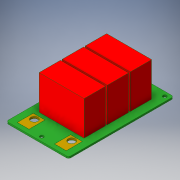
# Autodesk Inventor part: Cap_Platine
Saved by Autodesk Inventor 2016 (Build 200138000, 138)
## iProperties
Created: 2018-04-27
Part Number: Cap_Platine
Material: Generic
Document SubType Name: Modeling
Designer: Phil Erle
Density: 1 g/cm^3
Appearance: Smooth - Dark Forest Green
Author: Phil Erle
Autodesk Inventor part; units mm, degrees
ref_plane "YZ Plane" through (0, 0, 0) normal (1, 0, 0) x (0, 1, 0)
ref_plane "XZ Plane" through (0, 0, 0) normal (0, 1, 0) x (-1, 0, 0)
ref_plane "XY Plane" through (0, 0, 0) normal (0, 0, 1) x (1, 0, 0)
sketch "Sketch1" plane through (0, 0, 0) normal (0, 0, 1) x (1, 0, 0)
  line L0 (-29, -49) -> (29, -49)
  line L1 (29, -49) -> (29, 49)
  line L2 (29, 49) -> (-29, 49)
  line L3 (-29, 49) -> (-29, -49)
  line L4 (-29, -49) -> (29, 49) construction
  line L5 (29, -49) -> (-29, 49) construction
  point P0 (0, 0)
  dimension "d0" = 58
  dimension "d1" = 98
  constraints: 12 end point, 2 midpoint, 2 parallel, 1 horizontal, 1 perpendicular
  measures "d0" distance of L2.end L1.end
  measures "d1" distance of L1.end L0.end
extrude "Extrusion1" add sketch "Sketch1" along normal blind 1.6
sketch "Sketch2" plane through (0, 0, 1.6) normal (0, 0, 1) x (1, 0, 0)
  line L0 (-21, 16.5) -> (21, 16.5)
  line L1 (21, 16.5) -> (21, 36.5)
  line L2 (21, 36.5) -> (-21, 36.5)
  line L3 (-21, 36.5) -> (-21, 16.5)
  line L4 (-21, 16.5) -> (21, 36.5) construction
  line L5 (21, 16.5) -> (-21, 36.5) construction
  line L6 (-21, -5) -> (21, -5)
  line L7 (21, -5) -> (21, 15)
  line L8 (21, 15) -> (-21, 15)
  line L9 (-21, 15) -> (-21, -5)
  line L10 (-21, -5) -> (21, 15) construction
  line L11 (21, -5) -> (-21, 15) construction
  line L12 (-21, -26.5) -> (21, -26.5)
  line L13 (21, -26.5) -> (21, -6.5)
  line L14 (21, -6.5) -> (-21, -6.5)
  line L15 (-21, -6.5) -> (-21, -26.5)
  line L16 (-21, -26.5) -> (21, -6.5) construction
  line L17 (21, -26.5) -> (-21, -6.5) construction
  line L18 (-29, -49) -> (29, -49) projected
  line L19 (29, 49) -> (-29, 49) projected
  point P0 (0, 0)
  point P1 (0, 26.5)
  point P2 (0, 5)
  point P3 (0, -16.5)
  point P4 (0, 16.5)
  dimension "d4" = 42
  dimension "d5" = 20
  dimension "d6" = 20
  dimension "d7" = 20
  dimension "d8" = 1.5
  dimension "d9" = 1.5
  dimension "d31" = 12.5
  constraints: 36 end point, 7 midpoint, 6 parallel, 5 vertical alignment, 3 horizontal, 3 perpendicular
  measures "d4" distance of L1.end L2.end
  measures "d5" distance of L0.end L1.end
  measures "d6" distance of L6.end L7.end
  measures "d7" distance of L12.end L13.end
  measures "d8" distance of L13.end L6.end
  measures "d9" distance of L7.end L0.end
  measures "d31" distance between parallel lines of L19 L2
extrude "Extrusion2" add sketch "Sketch2" along normal blind 32
sketch "Sketch3" plane through (0, 0, 1.6) normal (0, 0, 1) x (1, 0, 0)
  line L0 (-24.75, -45) -> (24.75, -45) construction
  line L1 (24.75, -45) -> (24.75, 45) construction
  line L2 (24.75, 45) -> (-24.75, 45) construction
  line L3 (-24.75, 45) -> (-24.75, -45) construction
  line L4 (-24.75, -45) -> (24.75, 45) construction
  line L5 (24.75, -45) -> (-24.75, 45) construction
  point P0 (0, 0)
  point P1 (0, -45)
  dimension "d13" = 90
  dimension "d14" = 49.5
  constraints: 12 end point, 3 midpoint, 2 coincident, 2 parallel, 1 horizontal, 1 perpendicular
  measures "d13" distance of L2.end L0.start
  measures "d14" distance of L1.end L2.end
hole "Hole1" at (-24.75, 45, 1.6) at (24.75, 45, 1.6) at (0, -45, 1.6) direction (0, 0, -1) diameter 3.4 depth 9.525 tip angle 118 clearance for "Countersunk Flat Head Screw DIN EN ISO 2009" size "M3" standard "DIN"
fillet "Fillet1" radius 2 4 edges at (29, 49, 0.8) (-29, 49, 0.8) (29, -49, 0.8) (-29, -49, 0.8)
sketch "Sketch4" plane through (0, 0, 1.6) normal (0, 0, 1) x (1, 0, 0)
  line L0 (-17.375, -34.5) -> (17.375, -34.5) construction
  circle A0 centre (24.75, -45) radius 1.7 construction
  line L1 (-27, -49) -> (27, -49) projected
  point P0 (0, 0)
  point P1 (0, -34.5)
  dimension "d23" = 34.75
  dimension "d32" = 14.5
  constraints: 2 coincident, 2 end point, 1 horizontal, 1 midpoint, 1 vertical alignment
  measures "d23" distance of L0.start L0.end
  measures "d32" distance from line of L1 point (0, -34.5)
hole "Hole2" at (-17.375, -34.5, 1.6) at (17.375, -34.5, 1.6) direction (0, 0, -1) diameter 6.6 depth 9.525 tip angle 118 clearance for "Countersunk Flat Head Screw DIN EN ISO 2009" size "M6" standard "DIN"
sketch "Sketch5" plane through (0, 0, 1.6) normal (0, 0, 1) x (1, 0, 0)
  point P0 (0, 0)
sketch "Sketch6" plane through (0, 0, 1.6) normal (0, 0, 1) x (1, 0, 0)
  line L0 (-22.875, -45) -> (-11.875, -45)
  line L1 (-11.875, -45) -> (-11.875, -30)
  line L2 (-11.875, -30) -> (-22.875, -30)
  line L3 (-22.875, -30) -> (-22.875, -45)
  line L4 (-22.875, -45) -> (-11.875, -30) construction
  line L5 (-11.875, -45) -> (-22.875, -30) construction
  line L6 (11.875, -45) -> (22.875, -45)
  line L7 (22.875, -45) -> (22.875, -30)
  line L8 (22.875, -30) -> (11.875, -30)
  line L9 (11.875, -30) -> (11.875, -45)
  line L10 (11.875, -45) -> (22.875, -30) construction
  line L11 (22.875, -45) -> (11.875, -30) construction
  circle A0 centre (-17.375, -34.5) radius 3.3 projected
  circle A1 centre (17.375, -34.5) radius 3.3 projected
  point P0 (0, 0)
  point P1 (-17.375, -37.5)
  point P2 (17.375, -37.5)
  point P3 (-17.375, -37.5)
  point P4 (17.375, -37.5)
  dimension "d33" = 3
  dimension "d34" = 11
  dimension "d35" = 11
  dimension "d36" = 15
  constraints: 24 end point, 6 midpoint, 4 parallel, 2 horizontal, 2 perpendicular, 2 vertical alignment, 1 horizontal alignment, 1 point on line
  measures "d33" distance of A0.centre point (-17.375, -37.5)
  measures "d34" distance of L1.end L2.end
  measures "d35" distance of L7.end L8.end
  measures "d36" distance between parallel lines of L8 L6
extrude "Extrusion3" add sketch "Sketch6" along normal blind 0.1
body "Solid1"
